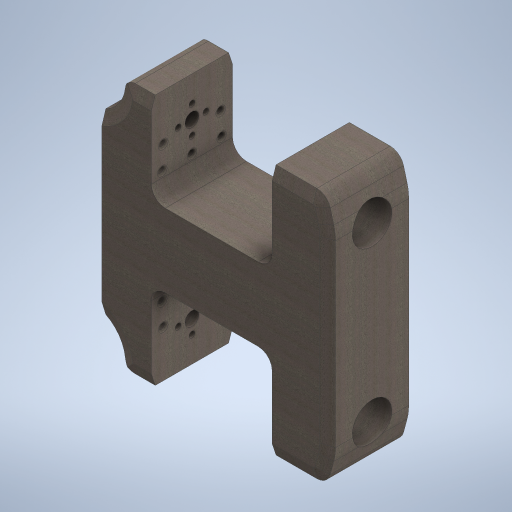
# Autodesk Inventor part: kadlub2_f
Saved by Autodesk Inventor 2023 (Build 270158000, 158)
## iProperties
Created: 2023-08-12
Part Number: kadlub2_f
Material: Steel
Document SubType Name: Modeling
Designer: Dawid
Density: 7.85 g/cm^3
Appearance: Walnut
Author: Dawid
Autodesk Inventor part; units mm, degrees
ref_plane "YZ Plane" through (0, 0, 0) normal (1, 0, 0) x (0, 1, 0)
ref_plane "XZ Plane" through (0, 0, 0) normal (0, 1, 0) x (-1, 0, 0)
ref_plane "XY Plane" through (0, 0, 0) normal (0, 0, 1) x (1, 0, 0)
sketch "Sketch3" plane through (0, 0, 0) normal (1, 0, 0) x (0, 1, 0)
  line L0 (85, 0) -> (85, -6)
  circle A0 centre (85, -6) radius 1.5
  circle A1 centre (73.5, -5.5) radius 1.5
  line L1 (21.5, 0) -> (68.5, -41) construction
  line L2 (68.5, 0) -> (21.5, -41) construction
  line L3 (68.5, -20.5) -> (73.5, -20.5)
  circle A2 centre (73.5, -20.5) radius 1.5
  circle A3 centre (88.5, -20.5) radius 10
  line L4 (73.5, -35.5) -> (73.5, -5.5)
  line L5 (73.5, -20.5) -> (73.5, -35.5)
  circle A4 centre (85, -35) radius 1.5
  circle A5 centre (73.5, -35.5) radius 1.5
  line L6 (98.5, 0) -> (98.5, -41)
  line L7 (68.5, 0) -> (68.5, -41)
  line L8 (90, -41) -> (90, 0)
  line L9 (90, 0) -> (90, -41)
  line L10 (85, -41) -> (85, -35)
  line L11 (88.5, -41) -> (88.5, 0)
  line L12 (78.5, 0) -> (78.5, -41)
  line L13 (98.5, -41) -> (88.5, -41)
  line L14 (90, -41) -> (85, -41)
  line L15 (11.5, 0) -> (78.5, -41) construction
  line L16 (78.5, 0) -> (11.5, -41) construction
  line L17 (90, -41) -> (0, -41)
  line L18 (90, 0) -> (0, -41) construction
  line L19 (0, -20.5) -> (90, -20.5)
  line L20 (90, -41) -> (0, -41)
  line L21 (0, 0) -> (90, -41) construction
  line L22 (-8.5, 0) -> (98.5, -41) construction
  line L23 (98.5, 0) -> (-8.5, -41) construction
  line L24 (98.5, -41) -> (-8.5, -41)
  line L25 (-8.5, 0) -> (98.5, 0)
  line L26 (0, 0) -> (90, 0)
  line L27 (0, 0) -> (90, 0)
  line L28 (21.5, 0) -> (68.5, 0)
  line L29 (11.5, 0) -> (78.5, 0)
  line L30 (78.5, -41) -> (11.5, -41)
  line L31 (68.5, -41) -> (21.5, -41)
  line L32 (11.5, -41) -> (11.5, 0)
  line L33 (0, -41) -> (0, 0)
  line L34 (0, 0) -> (0, -20.5)
  line L35 (0, -41) -> (0, 0)
  line L36 (-8.5, -41) -> (-8.5, 0)
  circle A6 centre (1.5, -20.5) radius 10
  line L37 (1.5, 0) -> (1.5, -41)
  line L38 (16.5, -41) -> (16.5, 0)
  line L39 (16.5, -35.5) -> (16.5, -5.5)
  circle A7 centre (16.5, -20.5) radius 1.5
  line L40 (16.5, -20.5) -> (16.5, -35.5)
  circle A8 centre (5, -35) radius 1.5
  line L41 (0, -41) -> (5, -41)
  line L42 (5, -41) -> (5, -35)
  line L43 (21.5, -41) -> (16.5, -41)
  circle A9 centre (16.5, -35.5) radius 1.5
  circle A10 centre (16.5, -5.5) radius 1.5
  circle A11 centre (5, -6) radius 1.5
  line L44 (5, 0) -> (5, -6)
  line L45 (0, 0) -> (5, 0)
  line L46 (-8.5, 0) -> (1.5, 0)
  line L47 (90, 0) -> (85, 0)
  line L48 (21.5, -41) -> (21.5, 0)
  line L49 (-8.5, 0) -> (-18.5, 0)
  point P0 (45, -38)
  point P1 (45, -38)
  point P2 (45, -20.5)
  point P3 (45, -20.5)
  dimension "d37" = 47
  dimension "d38" = 67
  dimension "d39" = 107
  dimension "d40" = 10
  dimension "d41" = 10
  dimension "d42" = 5
  dimension "d43" = 15
  dimension "d44" = 30
  dimension "d45" = 3
  dimension "d46" = 3
  dimension "d47" = 3
  dimension "d48" = 5
  dimension "d49" = 6
  dimension "d50" = 5
  dimension "d51" = 6
  dimension "d52" = 3
  dimension "d53" = 3
  dimension "d54" = 5
  dimension "d55" = 15
  dimension "d56" = 30
  dimension "d57" = 5
  dimension "d58" = 6
  dimension "d59" = 5
  dimension "d60" = 6
  dimension "d61" = 3
  dimension "d62" = 3
  dimension "d63" = 3
  dimension "d64" = 3
  dimension "d65" = 3
  dimension "d66" = 10
  constraints: 98 end point, 14 midpoint, 14 point on line, 12 centre point, 11 perpendicular, 10 coincident, 8 parallel, 4 horizontal, 1 tangent, 1 vertical, 7 other
  measures "d37" distance of L7.end L31.end
  measures "d38" distance of L12.end L30.end
  measures "d39" distance of L13.start L36.start
  measures "d40" distance of L36.end L37.start
  measures "d41" distance of L13.start L13.end
  measures "d42" distance of L31.end L43.end
  measures "d43" distance of L40.start L40.end
  measures "d44" distance of L40.end L39.end
  measures "d45" diameter of A10
  measures "d46" diameter of A9
  measures "d47" diameter of A7
  measures "d48" distance of L35.end L44.start
  measures "d49" distance of L44.start L44.end
  measures "d50" distance of L41.start L42.start
  measures "d51" distance of L42.start L42.end
  measures "d52" diameter of A8
  measures "d53" diameter of A11
  measures "d54" distance of L3.start L5.start
  measures "d55" distance of L5.start L4.start
  measures "d56" distance of L4.start L4.end
  measures "d57" distance of L47.start L47.end
  measures "d58" distance of L47.end L0.end
  measures "d59" distance of L14.start L10.start
  measures "d60" distance of L10.start L10.end
  measures "d61" diameter of A1
  measures "d62" diameter of A2
  measures "d63" diameter of A5
  measures "d64" diameter of A4
  measures "d65" diameter of A0
  measures "d66" distance of L36.end L49.end
extrude "Extrusion1" add sketch "Sketch3" along normal blind 10 contours L7 L25 L12 L19 A2 L3 | L19 L48 L25 L7 | L3 A2 L19 L12 L17 L7 | L7 L17 L48 L19 | L48 L17 L38 A9 A7 L19 | L19 A7 L38 A10 L25 L48 | L25 L11 A3 L12 | L12 A3 L11 L14 L17 | L38 A10 A7 L19 L32 L25 | L19 L11 A3 | A3 L11 L19 | L17 L32 L19 A7 L38 A9 | L32 A6 L37 L25 | L11 L25 L8 A3 | A3 L8 L19 L11 | L11 L19 L8 A3 | A3 L8 L13 L11 | L17 L37 A6 L32 | A6 L37 L19 | L19 L37 A6 | L37 A6 L33 L25 | L37 A6 L33 L19 | L19 L33 A6 L37 | L37 L17 L33 A6
sketch "Sketch15" plane through (10, 0, 0) normal (1, 0, 0) x (0, 0, -1)
  circle A0 centre (35, 85) radius 1.5 projected
  line L0 (35, 85) -> (33.5, 85)
  circle A1 centre (35.5, 73.5) radius 1.5 projected
  line L1 (35.5, 73.5) -> (34, 73.5)
  circle A2 centre (20.5, 73.5) radius 1.5 projected
  line L2 (20.5, 73.5) -> (19, 73.5)
  circle A3 centre (5.5, 73.5) radius 1.5 projected
  line L3 (5.5, 73.5) -> (4, 73.5)
  circle A4 centre (6, 85) radius 1.5 projected
  line L4 (6, 85) -> (4.5, 85)
  circle A5 centre (5.5, 16.5) radius 1.5 projected
  line L5 (5.5, 16.5) -> (4, 16.5)
  circle A6 centre (6, 5) radius 1.5 projected
  line L6 (6, 5) -> (4.5, 5)
  circle A7 centre (20.5, 16.5) radius 1.5 projected
  line L7 (20.5, 16.5) -> (19, 16.5)
  circle A8 centre (35.5, 16.5) radius 1.5 projected
  line L8 (35.5, 16.5) -> (34, 16.5)
  circle A9 centre (35, 5) radius 1.5 projected
  line L9 (35, 5) -> (33.5, 5)
  line L10 (41, 0) -> (41, 90) projected
  line L11 (41, 90) -> (0, 90)
  line L12 (0, 90) -> (0, 0)
  line L13 (0, 0) -> (41, 0)
  line L14 (41, 0) -> (41, 90)
  line L15 (20.5, 73.5) -> (20.5, 88.5)
  circle A10 centre (20.5, 88.5) radius 10
  line L16 (20.5, 98.5) -> (20.5, 108.5)
  line L17 (20.5, 108.5) -> (41, 108.5)
  line L18 (41, 108.5) -> (41, 90)
  line L19 (20.5, 108.5) -> (0, 108.5)
  line L20 (0, 90) -> (0, 0) projected
  line L21 (0, 108.5) -> (0, 90)
  line L22 (20.5, 16.5) -> (20.5, 1.5)
  circle A11 centre (20.5, 1.5) radius 10
  line L23 (20.5, -8.5) -> (20.5, -18.5)
  line L24 (20.5, -18.5) -> (0, -18.5)
  line L25 (0, -18.5) -> (0, 0)
  line L26 (0, 0) -> (41, 0) projected
  line L27 (41, 0) -> (41, -18.5)
  line L28 (41, -18.5) -> (20.5, -18.5)
  dimension "d217" = 20
  dimension "d220" = 20
  dimension "d216" = 15
  dimension "d218" = 10
  dimension "d219" = 15
  dimension "d221" = 10
  constraints: 52 end point, 10 horizontal alignment, 6 parallel, 6 point on line, 5 perpendicular, 4 vertical, 2 coincident, 2 collinear, 2 vertical alignment, 1 horizontal, 14 other
  measures "d216" distance of L2.start L15.end
  measures "d218" distance of L16.start L16.end
  measures "d219" distance of L7.start L22.end
  measures "d221" distance of L23.start L23.end
extrude "Extrusion9" add sketch "Sketch15" along normal blind 15
fillet "Fillet3" radius 18 2 edges at (10, 90, -20.5) (10, 0, -20.5)
sketch "Sketch16" plane through (25, 0, 0) normal (1, 0, 0) x (0, 0, -1)
  circle A0 centre (20.5, 73.5) radius 1.5 projected
  line L0 (20.5, 73.5) -> (20.5, 88.5)
  circle A1 centre (20.5, 16.5) radius 1.5 projected
  line L1 (20.5, 16.5) -> (20.5, 1.5)
  circle A2 centre (20.5, 88.5) radius 10
  circle A3 centre (20.5, 1.5) radius 10
  circle A4 centre (20.5, 88.5) radius 3.5
  circle A5 centre (20.5, 1.5) radius 3.5
  point P0 (0, 0)
  dimension "d225" = 15
  dimension "d226" = 15
  dimension "d227" = 20
  dimension "d228" = 20
  dimension "d229" = 7
  dimension "d230" = 7
  constraints: 4 centre point, 4 coincident, 4 end point, 2 vertical
  measures "d225" distance of L0.start L0.end
  measures "d226" distance of L1.start L1.end
  measures "d227" diameter of A2
  measures "d228" diameter of A3
  measures "d229" diameter of A4
  measures "d230" diameter of A5
extrude "Extrusion10" cut sketch "Sketch16" against normal blind 30 contours A4 | A5
fillet "Fillet4" radius 3.5 2 edges at (3.1579, 92, -20.5) (3.1579, -2, -20.5)
fillet "Fillet5" radius 1 10 edges at (25, 85, -33.5) (25, 73.5, -34) (25, 73.5, -19) (25, 73.5, -4) (25, 85, -4.5) (25, 16.5, -4) (25, 16.5, -19) (25, 5, -4.5) (25, 16.5, -34) (25, 5, -33.5)
sketch "Sketch17" plane through (25, 0, 0) normal (1, 0, 0) x (0, 0, -1)
  circle A0 centre (20.5, 88.5) radius 3.5 projected
  circle A1 centre (20.5, 88.5) radius 10
  circle A2 centre (20.5, 1.5) radius 3.5 projected
  circle A3 centre (20.5, 1.5) radius 10
  circle A4 centre (20.5, 88.5) radius 7
  circle A5 centre (20.5, 1.5) radius 7
  circle A6 centre (20.5, 95.5) radius 1.5
  circle A7 centre (20.5, 81.5) radius 1.5
  circle A8 centre (27.5, 88.5) radius 1.5
  circle A9 centre (13.5, 88.5) radius 1.5
  circle A10 centre (20.5, 8.5) radius 1.5
  circle A11 centre (13.5, 1.5) radius 1.5
  circle A12 centre (27.5, 1.5) radius 1.5
  circle A13 centre (20.5, -5.5) radius 1.5
  point P0 (0, 0)
  dimension "d235" = 20
  dimension "d236" = 20
  dimension "d237" = 14
  dimension "d238" = 14
  dimension "d239" = 3
  dimension "d240" = 3
  dimension "d241" = 3
  dimension "d242" = 3
  dimension "d243" = 3
  dimension "d244" = 3
  dimension "d245" = 3
  dimension "d246" = 3
  constraints: 12 centre point, 8 point on circle, 4 coincident
  measures "d235" diameter of A1
  measures "d236" diameter of A3
  measures "d237" diameter of A4
  measures "d238" diameter of A5
  measures "d239" diameter of A6
  measures "d240" diameter of A7
  measures "d241" diameter of A8
  measures "d242" diameter of A9
  measures "d243" diameter of A10
  measures "d244" diameter of A11
  measures "d245" diameter of A12
  measures "d246" diameter of A13
extrude "Extrusion11" cut sketch "Sketch17" against normal blind 8 contours A4 A8 | A4 A8 | A6 A4 | A4 A6 | A7 A4 | A4 A7 | A9 A4 | A4 A9 | A5 A12 | A5 A12 | A10 A5 | A5 A10 | A13 A5 | A5 A13 | A11 A5 | A5 A11
chamfer "Chamfer9" distance 6 distance2 2 4 edges at (7.2971, -6.6377, -41) (10, -17.3123, -41) (7.2971, 96.6377, -41) (10, 107.3123, -41) measured on face at (10.5, 107.3123, -41) measured on face at (7.722, 96.3742, -41) measured on face at (10.5, -17.3123, -41) measured on face at (7.722, -6.3742, -41)
chamfer "Chamfer10" distance 6 distance2 2 4 edges at (7.2971, -6.6377, 0) (10, -17.3123, 0) (7.2971, 96.6377, 0) (10, 107.3123, 0) measured on face at (7.722, 96.3742, 0) measured on face at (10.5, 107.3123, 0) measured on face at (10.5, -17.3123, 0) measured on face at (7.722, -6.3742, 0)
sketch "Sketch18" plane through (25, 0, 0) normal (1, 0, 0) x (0, 0, -1)
  line L0 (41, -18.5) -> (41, 108.5) projected
  line L1 (41, 108.5) -> (41, -18.5)
  line L2 (41, -18.5) -> (41, 45)
  line L3 (41, 45) -> (0, 45)
  line L4 (0, 83.4971) -> (0, 6.5029) projected
  circle A0 centre (20.5, 88.5) radius 3.5 projected
  circle A1 centre (20.5, 88.5) radius 10
  circle A2 centre (20.5, 1.5) radius 3.5 projected
  circle A3 centre (20.5, 1.5) radius 10
  line L5 (20.5, 1.5) -> (20.5, 26.5)
  arc A4 (17.1999, 87.3342) -> (23.8001, 87.3342) centre (20.5, 88.5) ccw projected
  line L6 (20.5, 88.5) -> (20.5, 63.5)
  line L7 (20.5, 63.5) -> (0, 63.5)
  line L8 (0, 63.5) -> (0, 26.5)
  line L9 (0, 26.5) -> (41, 26.5)
  line L10 (20.5, 63.5) -> (41, 63.5)
  point P0 (0, 0)
  dimension "d255" = 20
  dimension "d256" = 20
  dimension "d257" = 25
  dimension "d258" = 25
  constraints: 18 end point, 5 point on line, 3 vertical, 2 centre point, 2 coincident, 2 midpoint, 2 perpendicular
  measures "d255" diameter of A1
  measures "d256" diameter of A3
  measures "d257" distance of L5.start L5.end
  measures "d258" distance of L6.start L6.end
extrude "Extrusion12" add sketch "Sketch18" along normal blind 61 contours L9 L4 L3 L0 | L3 L4 L7 L10 L0
fillet "Fillet6" radius 7 2 edges at (25, 63.5, -20.5) (25, 26.5, -20.5)
sketch "Sketch19" plane through (86, 0, 0) normal (1, 0, 0) x (0, 0, -1)
  line L0 (41, 70.5) -> (41, 108.5) projected
  line L1 (41, 108.5) -> (0, 108.5)
  line L2 (0, 108.5) -> (0, -18.5)
  line L3 (0, -18.5) -> (41, -18.5)
  line L4 (41, -18.5) -> (41, 108.5)
  circle A0 centre (20.5, 88.5) radius 3.5 projected
  circle A1 centre (20.5, 88.5) radius 10
  circle A2 centre (20.5, 1.5) radius 3.5 projected
  circle A3 centre (20.5, 1.5) radius 10
  point P0 (0, 0)
  dimension "d262" = 20
  dimension "d263" = 20
  constraints: 8 end point, 2 centre point, 2 coincident, 2 parallel, 1 horizontal, 1 perpendicular
  measures "d262" diameter of A1
  measures "d263" diameter of A3
extrude "Extrusion13" add sketch "Sketch19" along normal blind 30 contours L4 L3 L2 L1 L0
fillet "Fillet7" radius 7 2 edges at (86, 26.5, -20.5) (86, 63.5, -20.5)
chamfer "Chamfer11" distance 15 distance2 4 2 edges at (116, 108.5, -20.5) (116, -18.5, -20.5) measured on face at (116, 108, -20.5) measured on face at (116, -18, -20.5)
fillet "Fillet8" radius 25 4 edges at (116, 93.5, -35.0801) (116, 93.5, -5.9199) (116, -3.5, -35.0801) (116, -3.5, -5.9199)
fillet "Fillet9" radius 7 2 edges at (112, 108.5, -20.5) (112, -18.5, -20.5)
chamfer "Chamfer12" distance 6 distance2 2 11 edges at (20.5, 108.5, -41) (96.311, 108.5, -41) (110.8867, 107.0509, -41) (114.2708, 99.9846, -41) (115.7881, 93.4722, -41) (116, 45, -41) (115.7881, -3.4722, -41) (114.2708, -9.9846, -41) (110.8867, -17.0509, -41) (96.311, -18.5, -41) (20.5, -18.5, -41) measured on face at (115.5, 45, -41) measured on face at (115.2923, 93.4073, -41) measured on face at (96.311, -18, -41) measured on face at (20.5, -18, -41) measured on face at (96.311, 108, -41) measured on face at (110.5821, 106.6544, -41) measured on face at (113.7877, 99.8557, -41) measured on face at (115.2923, -3.4073, -41) measured on face at (110.5821, -16.6544, -41) measured on face at (20.5, 108, -41) measured on face at (113.7877, -9.8557, -41)
chamfer "Chamfer13" distance 6 distance2 2 11 edges at (116, 45, 0) (115.7881, -3.4722, 0) (114.2708, -9.9846, 0) (110.8867, -17.0509, 0) (96.311, -18.5, 0) (115.7881, 93.4722, 0) (114.2708, 99.9846, 0) (110.8867, 107.0509, 0) (96.311, 108.5, 0) (20.5, 108.5, 0) (20.5, -18.5, 0) measured on face at (110.5821, -16.6544, 0) measured on face at (20.5, 108, 0) measured on face at (115.5, 45, 0) measured on face at (96.311, -18, 0) measured on face at (115.2923, 93.4073, 0) measured on face at (110.5821, 106.6544, 0) measured on face at (20.5, -18, 0) measured on face at (115.2923, -3.4073, 0) measured on face at (96.311, 108, 0) measured on face at (113.7877, 99.8557, 0) measured on face at (113.7877, -9.8557, 0)
fillet "Fillet10" radius 5 2 edges at (10, -18.5, -20.5) (10, 108.5, -20.5)
body "Solid1"
